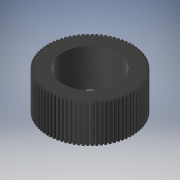
# Autodesk Inventor part: タミヤダンパー部品3
Saved by Autodesk Inventor 2020.1 (Build 241239000, 239)
## iProperties
Created: 2018-09-17
Part Number: タミヤダンパー部品3
Material: アセタール樹脂、黒
Document SubType Name: Modeling
Designer: 杉本　賢二郎
Density: 1.425 g/cm^3
Appearance: 滑らか - 黒
Author: 杉本　賢二郎
Autodesk Inventor part; units mm, degrees
ref_plane "YZ Plane" through (0, 0, 0) normal (1, 0, 0) x (0, 1, 0)
ref_plane "XZ Plane" through (0, 0, 0) normal (0, 1, 0) x (-1, 0, 0)
ref_plane "XY Plane" through (0, 0, 0) normal (0, 0, 1) x (1, 0, 0)
sketch "スケッチ1" plane through (0, 0, 0) normal (0, 1, 0) x (-1, 0, 0)
  arc A0 (0.0974, 4.9991) -> (-0.0974, 4.9991) centre (0, 0) ccw
  arc A1 (0.05, 4.8047) -> (-0.05, 4.8047) centre (0, 0) ccw
  line L0 (0.05, 4.8047) -> (0.0974, 4.9991)
  line L1 (-0.05, 4.8047) -> (-0.0974, 4.9991)
  line L2 (0, 4.9011) -> (0, 0)
  line L3 (-0.4268, 4.786) -> (-0.4893, 4.976)
  arc A2 (-0.2952, 4.9913) -> (-0.4893, 4.976) centre (0, 0) ccw
  line L4 (-0.3271, 4.7939) -> (-0.2952, 4.9913)
  arc A3 (-0.3271, 4.7939) -> (-0.4268, 4.786) centre (0, 0) ccw
  line L5 (-0.801, 4.7378) -> (-0.8782, 4.9223)
  arc A4 (-0.6859, 4.9527) -> (-0.8782, 4.9223) centre (0, 0) ccw
  line L6 (-0.7022, 4.7534) -> (-0.6859, 4.9527)
  arc A5 (-0.7022, 4.7534) -> (-0.801, 4.7378) centre (0, 0) ccw
  line L7 (-1.1703, 4.6603) -> (-1.2617, 4.8382)
  arc A6 (-1.0723, 4.8837) -> (-1.2617, 4.8382) centre (0, 0) ccw
  line L8 (-1.073, 4.6837) -> (-1.0723, 4.8837)
  arc A7 (-1.073, 4.6837) -> (-1.1703, 4.6603) centre (0, 0) ccw
  line L9 (-1.5323, 4.5541) -> (-1.6374, 4.7243)
  arc A8 (-1.4522, 4.7845) -> (-1.6374, 4.7243) centre (0, 0) ccw
  line L10 (-1.4372, 4.585) -> (-1.4522, 4.7845)
  arc A9 (-1.4372, 4.585) -> (-1.5323, 4.5541) centre (0, 0) ccw
  line L11 (-1.8849, 4.4199) -> (-2.003, 4.5813)
  arc A10 (-1.8231, 4.6558) -> (-2.003, 4.5813) centre (0, 0) ccw
  line L12 (-1.7925, 4.4581) -> (-1.8231, 4.6558)
  arc A11 (-1.7925, 4.4581) -> (-1.8849, 4.4199) centre (0, 0) ccw
  line L13 (-2.2259, 4.2584) -> (-2.3563, 4.41)
  arc A12 (-2.1828, 4.4984) -> (-2.3563, 4.41) centre (0, 0) ccw
  line L14 (-2.1368, 4.3038) -> (-2.1828, 4.4984)
  arc A13 (-2.1368, 4.3038) -> (-2.2259, 4.2584) centre (0, 0) ccw
  line L15 (-2.5531, 4.0706) -> (-2.695, 4.2115)
  arc A14 (-2.529, 4.3133) -> (-2.695, 4.2115) centre (0, 0) ccw
  line L16 (-2.4678, 4.1228) -> (-2.529, 4.3133)
  arc A15 (-2.4678, 4.1228) -> (-2.5531, 4.0706) centre (0, 0) ccw
  line L17 (-2.8646, 3.8577) -> (-3.0171, 3.9871)
  arc A16 (-2.8596, 4.1015) -> (-3.0171, 3.9871) centre (0, 0) ccw
  line L18 (-2.7837, 3.9165) -> (-2.8596, 4.1015)
  arc A17 (-2.7837, 3.9165) -> (-2.8646, 3.8577) centre (0, 0) ccw
  line L19 (-3.1584, 3.6211) -> (-3.3207, 3.7381)
  arc A18 (-3.1726, 3.8645) -> (-3.3207, 3.7381) centre (0, 0) ccw
  line L20 (-3.0824, 3.686) -> (-3.1726, 3.8645)
  arc A19 (-3.0824, 3.686) -> (-3.1584, 3.6211) centre (0, 0) ccw
  line L21 (-3.4328, 3.3621) -> (-3.6037, 3.466)
  arc A20 (-3.466, 3.6037) -> (-3.6037, 3.466) centre (0, 0) ccw
  line L22 (-3.3621, 3.4328) -> (-3.466, 3.6037)
  arc A21 (-3.3621, 3.4328) -> (-3.4328, 3.3621) centre (0, 0) ccw
  line L23 (-3.686, 3.0824) -> (-3.8645, 3.1726)
  arc A22 (-3.7381, 3.3207) -> (-3.8645, 3.1726) centre (0, 0) ccw
  line L24 (-3.6211, 3.1584) -> (-3.7381, 3.3207)
  arc A23 (-3.6211, 3.1584) -> (-3.686, 3.0824) centre (0, 0) ccw
  line L25 (-3.9165, 2.7837) -> (-4.1015, 2.8596)
  arc A24 (-3.9871, 3.0171) -> (-4.1015, 2.8596) centre (0, 0) ccw
  line L26 (-3.8577, 2.8646) -> (-3.9871, 3.0171)
  arc A25 (-3.8577, 2.8646) -> (-3.9165, 2.7837) centre (0, 0) ccw
  line L27 (-4.1228, 2.4678) -> (-4.3133, 2.529)
  arc A26 (-4.2115, 2.695) -> (-4.3133, 2.529) centre (0, 0) ccw
  line L28 (-4.0706, 2.5531) -> (-4.2115, 2.695)
  arc A27 (-4.0706, 2.5531) -> (-4.1228, 2.4678) centre (0, 0) ccw
  line L29 (-4.3038, 2.1368) -> (-4.4984, 2.1828)
  arc A28 (-4.41, 2.3563) -> (-4.4984, 2.1828) centre (0, 0) ccw
  line L30 (-4.2584, 2.2259) -> (-4.41, 2.3563)
  arc A29 (-4.2584, 2.2259) -> (-4.3038, 2.1368) centre (0, 0) ccw
  line L31 (-4.4581, 1.7925) -> (-4.6558, 1.8231)
  arc A30 (-4.5813, 2.003) -> (-4.6558, 1.8231) centre (0, 0) ccw
  line L32 (-4.4199, 1.8849) -> (-4.5813, 2.003)
  arc A31 (-4.4199, 1.8849) -> (-4.4581, 1.7925) centre (0, 0) ccw
  line L33 (-4.585, 1.4372) -> (-4.7845, 1.4522)
  arc A32 (-4.7243, 1.6374) -> (-4.7845, 1.4522) centre (0, 0) ccw
  line L34 (-4.5541, 1.5323) -> (-4.7243, 1.6374)
  arc A33 (-4.5541, 1.5323) -> (-4.585, 1.4372) centre (0, 0) ccw
  line L35 (-4.6837, 1.073) -> (-4.8837, 1.0723)
  arc A34 (-4.8382, 1.2617) -> (-4.8837, 1.0723) centre (0, 0) ccw
  line L36 (-4.6603, 1.1703) -> (-4.8382, 1.2617)
  arc A35 (-4.6603, 1.1703) -> (-4.6837, 1.073) centre (0, 0) ccw
  line L37 (-4.7534, 0.7022) -> (-4.9527, 0.6859)
  arc A36 (-4.9223, 0.8782) -> (-4.9527, 0.6859) centre (0, 0) ccw
  line L38 (-4.7378, 0.801) -> (-4.9223, 0.8782)
  arc A37 (-4.7378, 0.801) -> (-4.7534, 0.7022) centre (0, 0) ccw
  line L39 (-4.7939, 0.3271) -> (-4.9913, 0.2952)
  arc A38 (-4.976, 0.4893) -> (-4.9913, 0.2952) centre (0, 0) ccw
  line L40 (-4.786, 0.4268) -> (-4.976, 0.4893)
  arc A39 (-4.786, 0.4268) -> (-4.7939, 0.3271) centre (0, 0) ccw
  line L41 (-4.8047, -0.05) -> (-4.9991, -0.0974)
  arc A40 (-4.9991, 0.0974) -> (-4.9991, -0.0974) centre (0, 0) ccw
  line L42 (-4.8047, 0.05) -> (-4.9991, 0.0974)
  arc A41 (-4.8047, 0.05) -> (-4.8047, -0.05) centre (0, 0) ccw
  line L43 (-4.786, -0.4268) -> (-4.976, -0.4893)
  arc A42 (-4.9913, -0.2952) -> (-4.976, -0.4893) centre (0, 0) ccw
  line L44 (-4.7939, -0.3271) -> (-4.9913, -0.2952)
  arc A43 (-4.7939, -0.3271) -> (-4.786, -0.4268) centre (0, 0) ccw
  line L45 (-4.7378, -0.801) -> (-4.9223, -0.8782)
  arc A44 (-4.9527, -0.6859) -> (-4.9223, -0.8782) centre (0, 0) ccw
  line L46 (-4.7534, -0.7022) -> (-4.9527, -0.6859)
  arc A45 (-4.7534, -0.7022) -> (-4.7378, -0.801) centre (0, 0) ccw
  line L47 (-4.6603, -1.1703) -> (-4.8382, -1.2617)
  arc A46 (-4.8837, -1.0723) -> (-4.8382, -1.2617) centre (0, 0) ccw
  line L48 (-4.6837, -1.073) -> (-4.8837, -1.0723)
  arc A47 (-4.6837, -1.073) -> (-4.6603, -1.1703) centre (0, 0) ccw
  line L49 (-4.5541, -1.5323) -> (-4.7243, -1.6374)
  arc A48 (-4.7845, -1.4522) -> (-4.7243, -1.6374) centre (0, 0) ccw
  line L50 (-4.585, -1.4372) -> (-4.7845, -1.4522)
  arc A49 (-4.585, -1.4372) -> (-4.5541, -1.5323) centre (0, 0) ccw
  line L51 (-4.4199, -1.8849) -> (-4.5813, -2.003)
  arc A50 (-4.6558, -1.8231) -> (-4.5813, -2.003) centre (0, 0) ccw
  line L52 (-4.4581, -1.7925) -> (-4.6558, -1.8231)
  arc A51 (-4.4581, -1.7925) -> (-4.4199, -1.8849) centre (0, 0) ccw
  line L53 (-4.2584, -2.2259) -> (-4.41, -2.3563)
  arc A52 (-4.4984, -2.1828) -> (-4.41, -2.3563) centre (0, 0) ccw
  line L54 (-4.3038, -2.1368) -> (-4.4984, -2.1828)
  arc A53 (-4.3038, -2.1368) -> (-4.2584, -2.2259) centre (0, 0) ccw
  line L55 (-4.0706, -2.5531) -> (-4.2115, -2.695)
  arc A54 (-4.3133, -2.529) -> (-4.2115, -2.695) centre (0, 0) ccw
  line L56 (-4.1228, -2.4678) -> (-4.3133, -2.529)
  arc A55 (-4.1228, -2.4678) -> (-4.0706, -2.5531) centre (0, 0) ccw
  line L57 (-3.8577, -2.8646) -> (-3.9871, -3.0171)
  arc A56 (-4.1015, -2.8596) -> (-3.9871, -3.0171) centre (0, 0) ccw
  line L58 (-3.9165, -2.7837) -> (-4.1015, -2.8596)
  arc A57 (-3.9165, -2.7837) -> (-3.8577, -2.8646) centre (0, 0) ccw
  line L59 (-3.6211, -3.1584) -> (-3.7381, -3.3207)
  arc A58 (-3.8645, -3.1726) -> (-3.7381, -3.3207) centre (0, 0) ccw
  line L60 (-3.686, -3.0824) -> (-3.8645, -3.1726)
  arc A59 (-3.686, -3.0824) -> (-3.6211, -3.1584) centre (0, 0) ccw
  line L61 (-3.3621, -3.4328) -> (-3.466, -3.6037)
  arc A60 (-3.6037, -3.466) -> (-3.466, -3.6037) centre (0, 0) ccw
  line L62 (-3.4328, -3.3621) -> (-3.6037, -3.466)
  arc A61 (-3.4328, -3.3621) -> (-3.3621, -3.4328) centre (0, 0) ccw
  line L63 (-3.0824, -3.686) -> (-3.1726, -3.8645)
  arc A62 (-3.3207, -3.7381) -> (-3.1726, -3.8645) centre (0, 0) ccw
  line L64 (-3.1584, -3.6211) -> (-3.3207, -3.7381)
  arc A63 (-3.1584, -3.6211) -> (-3.0824, -3.686) centre (0, 0) ccw
  line L65 (-2.7837, -3.9165) -> (-2.8596, -4.1015)
  arc A64 (-3.0171, -3.9871) -> (-2.8596, -4.1015) centre (0, 0) ccw
  line L66 (-2.8646, -3.8577) -> (-3.0171, -3.9871)
  arc A65 (-2.8646, -3.8577) -> (-2.7837, -3.9165) centre (0, 0) ccw
  line L67 (-2.4678, -4.1228) -> (-2.529, -4.3133)
  arc A66 (-2.695, -4.2115) -> (-2.529, -4.3133) centre (0, 0) ccw
  line L68 (-2.5531, -4.0706) -> (-2.695, -4.2115)
  arc A67 (-2.5531, -4.0706) -> (-2.4678, -4.1228) centre (0, 0) ccw
  line L69 (-2.1368, -4.3038) -> (-2.1828, -4.4984)
  arc A68 (-2.3563, -4.41) -> (-2.1828, -4.4984) centre (0, 0) ccw
  line L70 (-2.2259, -4.2584) -> (-2.3563, -4.41)
  arc A69 (-2.2259, -4.2584) -> (-2.1368, -4.3038) centre (0, 0) ccw
  line L71 (-1.7925, -4.4581) -> (-1.8231, -4.6558)
  arc A70 (-2.003, -4.5813) -> (-1.8231, -4.6558) centre (0, 0) ccw
  line L72 (-1.8849, -4.4199) -> (-2.003, -4.5813)
  arc A71 (-1.8849, -4.4199) -> (-1.7925, -4.4581) centre (0, 0) ccw
  line L73 (-1.4372, -4.585) -> (-1.4522, -4.7845)
  arc A72 (-1.6374, -4.7243) -> (-1.4522, -4.7845) centre (0, 0) ccw
  line L74 (-1.5323, -4.5541) -> (-1.6374, -4.7243)
  arc A73 (-1.5323, -4.5541) -> (-1.4372, -4.585) centre (0, 0) ccw
  line L75 (-1.073, -4.6837) -> (-1.0723, -4.8837)
  arc A74 (-1.2617, -4.8382) -> (-1.0723, -4.8837) centre (0, 0) ccw
  line L76 (-1.1703, -4.6603) -> (-1.2617, -4.8382)
  arc A75 (-1.1703, -4.6603) -> (-1.073, -4.6837) centre (0, 0) ccw
  line L77 (-0.7022, -4.7534) -> (-0.6859, -4.9527)
  arc A76 (-0.8782, -4.9223) -> (-0.6859, -4.9527) centre (0, 0) ccw
  line L78 (-0.801, -4.7378) -> (-0.8782, -4.9223)
  arc A77 (-0.801, -4.7378) -> (-0.7022, -4.7534) centre (0, 0) ccw
  line L79 (-0.3271, -4.7939) -> (-0.2952, -4.9913)
  arc A78 (-0.4893, -4.976) -> (-0.2952, -4.9913) centre (0, 0) ccw
  line L80 (-0.4268, -4.786) -> (-0.4893, -4.976)
  arc A79 (-0.4268, -4.786) -> (-0.3271, -4.7939) centre (0, 0) ccw
  line L81 (0.05, -4.8047) -> (0.0974, -4.9991)
  arc A80 (-0.0974, -4.9991) -> (0.0974, -4.9991) centre (0, 0) ccw
  line L82 (-0.05, -4.8047) -> (-0.0974, -4.9991)
  arc A81 (-0.05, -4.8047) -> (0.05, -4.8047) centre (0, 0) ccw
  line L83 (0.4268, -4.786) -> (0.4893, -4.976)
  arc A82 (0.2952, -4.9913) -> (0.4893, -4.976) centre (0, 0) ccw
  line L84 (0.3271, -4.7939) -> (0.2952, -4.9913)
  arc A83 (0.3271, -4.7939) -> (0.4268, -4.786) centre (0, 0) ccw
  line L85 (0.801, -4.7378) -> (0.8782, -4.9223)
  arc A84 (0.6859, -4.9527) -> (0.8782, -4.9223) centre (0, 0) ccw
  line L86 (0.7022, -4.7534) -> (0.6859, -4.9527)
  arc A85 (0.7022, -4.7534) -> (0.801, -4.7378) centre (0, 0) ccw
  line L87 (1.1703, -4.6603) -> (1.2617, -4.8382)
  arc A86 (1.0723, -4.8837) -> (1.2617, -4.8382) centre (0, 0) ccw
  line L88 (1.073, -4.6837) -> (1.0723, -4.8837)
  arc A87 (1.073, -4.6837) -> (1.1703, -4.6603) centre (0, 0) ccw
  line L89 (1.5323, -4.5541) -> (1.6374, -4.7243)
  arc A88 (1.4522, -4.7845) -> (1.6374, -4.7243) centre (0, 0) ccw
  line L90 (1.4372, -4.585) -> (1.4522, -4.7845)
  arc A89 (1.4372, -4.585) -> (1.5323, -4.5541) centre (0, 0) ccw
  line L91 (1.8849, -4.4199) -> (2.003, -4.5813)
  arc A90 (1.8231, -4.6558) -> (2.003, -4.5813) centre (0, 0) ccw
  line L92 (1.7925, -4.4581) -> (1.8231, -4.6558)
  arc A91 (1.7925, -4.4581) -> (1.8849, -4.4199) centre (0, 0) ccw
  line L93 (2.2259, -4.2584) -> (2.3563, -4.41)
  arc A92 (2.1828, -4.4984) -> (2.3563, -4.41) centre (0, 0) ccw
  line L94 (2.1368, -4.3038) -> (2.1828, -4.4984)
  arc A93 (2.1368, -4.3038) -> (2.2259, -4.2584) centre (0, 0) ccw
  line L95 (2.5531, -4.0706) -> (2.695, -4.2115)
  arc A94 (2.529, -4.3133) -> (2.695, -4.2115) centre (0, 0) ccw
  line L96 (2.4678, -4.1228) -> (2.529, -4.3133)
  arc A95 (2.4678, -4.1228) -> (2.5531, -4.0706) centre (0, 0) ccw
  line L97 (2.8646, -3.8577) -> (3.0171, -3.9871)
  arc A96 (2.8596, -4.1015) -> (3.0171, -3.9871) centre (0, 0) ccw
  line L98 (2.7837, -3.9165) -> (2.8596, -4.1015)
  arc A97 (2.7837, -3.9165) -> (2.8646, -3.8577) centre (0, 0) ccw
  line L99 (3.1584, -3.6211) -> (3.3207, -3.7381)
  arc A98 (3.1726, -3.8645) -> (3.3207, -3.7381) centre (0, 0) ccw
  line L100 (3.0824, -3.686) -> (3.1726, -3.8645)
  arc A99 (3.0824, -3.686) -> (3.1584, -3.6211) centre (0, 0) ccw
  line L101 (3.4328, -3.3621) -> (3.6037, -3.466)
  arc A100 (3.466, -3.6037) -> (3.6037, -3.466) centre (0, 0) ccw
  line L102 (3.3621, -3.4328) -> (3.466, -3.6037)
  arc A101 (3.3621, -3.4328) -> (3.4328, -3.3621) centre (0, 0) ccw
  line L103 (3.686, -3.0824) -> (3.8645, -3.1726)
  arc A102 (3.7381, -3.3207) -> (3.8645, -3.1726) centre (0, 0) ccw
  line L104 (3.6211, -3.1584) -> (3.7381, -3.3207)
  arc A103 (3.6211, -3.1584) -> (3.686, -3.0824) centre (0, 0) ccw
  line L105 (3.9165, -2.7837) -> (4.1015, -2.8596)
  arc A104 (3.9871, -3.0171) -> (4.1015, -2.8596) centre (0, 0) ccw
  line L106 (3.8577, -2.8646) -> (3.9871, -3.0171)
  arc A105 (3.8577, -2.8646) -> (3.9165, -2.7837) centre (0, 0) ccw
  line L107 (4.1228, -2.4678) -> (4.3133, -2.529)
  arc A106 (4.2115, -2.695) -> (4.3133, -2.529) centre (0, 0) ccw
  line L108 (4.0706, -2.5531) -> (4.2115, -2.695)
  arc A107 (4.0706, -2.5531) -> (4.1228, -2.4678) centre (0, 0) ccw
  line L109 (4.3038, -2.1368) -> (4.4984, -2.1828)
  arc A108 (4.41, -2.3563) -> (4.4984, -2.1828) centre (0, 0) ccw
  line L110 (4.2584, -2.2259) -> (4.41, -2.3563)
  arc A109 (4.2584, -2.2259) -> (4.3038, -2.1368) centre (0, 0) ccw
  line L111 (4.4581, -1.7925) -> (4.6558, -1.8231)
  arc A110 (4.5813, -2.003) -> (4.6558, -1.8231) centre (0, 0) ccw
  line L112 (4.4199, -1.8849) -> (4.5813, -2.003)
  arc A111 (4.4199, -1.8849) -> (4.4581, -1.7925) centre (0, 0) ccw
  line L113 (4.585, -1.4372) -> (4.7845, -1.4522)
  arc A112 (4.7243, -1.6374) -> (4.7845, -1.4522) centre (0, 0) ccw
  line L114 (4.5541, -1.5323) -> (4.7243, -1.6374)
  arc A113 (4.5541, -1.5323) -> (4.585, -1.4372) centre (0, 0) ccw
  line L115 (4.6837, -1.073) -> (4.8837, -1.0723)
  arc A114 (4.8382, -1.2617) -> (4.8837, -1.0723) centre (0, 0) ccw
  line L116 (4.6603, -1.1703) -> (4.8382, -1.2617)
  arc A115 (4.6603, -1.1703) -> (4.6837, -1.073) centre (0, 0) ccw
  line L117 (4.7534, -0.7022) -> (4.9527, -0.6859)
  arc A116 (4.9223, -0.8782) -> (4.9527, -0.6859) centre (0, 0) ccw
  line L118 (4.7378, -0.801) -> (4.9223, -0.8782)
  arc A117 (4.7378, -0.801) -> (4.7534, -0.7022) centre (0, 0) ccw
  line L119 (4.7939, -0.3271) -> (4.9913, -0.2952)
  arc A118 (4.976, -0.4893) -> (4.9913, -0.2952) centre (0, 0) ccw
  line L120 (4.786, -0.4268) -> (4.976, -0.4893)
  arc A119 (4.786, -0.4268) -> (4.7939, -0.3271) centre (0, 0) ccw
  line L121 (4.8047, 0.05) -> (4.9991, 0.0974)
  arc A120 (4.9991, -0.0974) -> (4.9991, 0.0974) centre (0, 0) ccw
  line L122 (4.8047, -0.05) -> (4.9991, -0.0974)
  arc A121 (4.8047, -0.05) -> (4.8047, 0.05) centre (0, 0) ccw
  line L123 (4.786, 0.4268) -> (4.976, 0.4893)
  arc A122 (4.9913, 0.2952) -> (4.976, 0.4893) centre (0, 0) ccw
  line L124 (4.7939, 0.3271) -> (4.9913, 0.2952)
  arc A123 (4.7939, 0.3271) -> (4.786, 0.4268) centre (0, 0) ccw
  line L125 (4.7378, 0.801) -> (4.9223, 0.8782)
  arc A124 (4.9527, 0.6859) -> (4.9223, 0.8782) centre (0, 0) ccw
  line L126 (4.7534, 0.7022) -> (4.9527, 0.6859)
  arc A125 (4.7534, 0.7022) -> (4.7378, 0.801) centre (0, 0) ccw
  line L127 (4.6603, 1.1703) -> (4.8382, 1.2617)
  arc A126 (4.8837, 1.0723) -> (4.8382, 1.2617) centre (0, 0) ccw
  line L128 (4.6837, 1.073) -> (4.8837, 1.0723)
  arc A127 (4.6837, 1.073) -> (4.6603, 1.1703) centre (0, 0) ccw
  line L129 (4.5541, 1.5323) -> (4.7243, 1.6374)
  arc A128 (4.7845, 1.4522) -> (4.7243, 1.6374) centre (0, 0) ccw
  line L130 (4.585, 1.4372) -> (4.7845, 1.4522)
  arc A129 (4.585, 1.4372) -> (4.5541, 1.5323) centre (0, 0) ccw
  line L131 (4.4199, 1.8849) -> (4.5813, 2.003)
  arc A130 (4.6558, 1.8231) -> (4.5813, 2.003) centre (0, 0) ccw
  line L132 (4.4581, 1.7925) -> (4.6558, 1.8231)
  arc A131 (4.4581, 1.7925) -> (4.4199, 1.8849) centre (0, 0) ccw
  line L133 (4.2584, 2.2259) -> (4.41, 2.3563)
  arc A132 (4.4984, 2.1828) -> (4.41, 2.3563) centre (0, 0) ccw
  line L134 (4.3038, 2.1368) -> (4.4984, 2.1828)
  arc A133 (4.3038, 2.1368) -> (4.2584, 2.2259) centre (0, 0) ccw
  line L135 (4.0706, 2.5531) -> (4.2115, 2.695)
  arc A134 (4.3133, 2.529) -> (4.2115, 2.695) centre (0, 0) ccw
  line L136 (4.1228, 2.4678) -> (4.3133, 2.529)
  arc A135 (4.1228, 2.4678) -> (4.0706, 2.5531) centre (0, 0) ccw
  line L137 (3.8577, 2.8646) -> (3.9871, 3.0171)
  arc A136 (4.1015, 2.8596) -> (3.9871, 3.0171) centre (0, 0) ccw
  line L138 (3.9165, 2.7837) -> (4.1015, 2.8596)
  arc A137 (3.9165, 2.7837) -> (3.8577, 2.8646) centre (0, 0) ccw
  line L139 (3.6211, 3.1584) -> (3.7381, 3.3207)
  arc A138 (3.8645, 3.1726) -> (3.7381, 3.3207) centre (0, 0) ccw
  line L140 (3.686, 3.0824) -> (3.8645, 3.1726)
  arc A139 (3.686, 3.0824) -> (3.6211, 3.1584) centre (0, 0) ccw
  line L141 (3.3621, 3.4328) -> (3.466, 3.6037)
  arc A140 (3.6037, 3.466) -> (3.466, 3.6037) centre (0, 0) ccw
  line L142 (3.4328, 3.3621) -> (3.6037, 3.466)
  arc A141 (3.4328, 3.3621) -> (3.3621, 3.4328) centre (0, 0) ccw
  line L143 (3.0824, 3.686) -> (3.1726, 3.8645)
  arc A142 (3.3207, 3.7381) -> (3.1726, 3.8645) centre (0, 0) ccw
  line L144 (3.1584, 3.6211) -> (3.3207, 3.7381)
  arc A143 (3.1584, 3.6211) -> (3.0824, 3.686) centre (0, 0) ccw
  line L145 (2.7837, 3.9165) -> (2.8596, 4.1015)
  arc A144 (3.0171, 3.9871) -> (2.8596, 4.1015) centre (0, 0) ccw
  line L146 (2.8646, 3.8577) -> (3.0171, 3.9871)
  arc A145 (2.8646, 3.8577) -> (2.7837, 3.9165) centre (0, 0) ccw
  line L147 (2.4678, 4.1228) -> (2.529, 4.3133)
  arc A146 (2.695, 4.2115) -> (2.529, 4.3133) centre (0, 0) ccw
  line L148 (2.5531, 4.0706) -> (2.695, 4.2115)
  arc A147 (2.5531, 4.0706) -> (2.4678, 4.1228) centre (0, 0) ccw
  line L149 (2.1368, 4.3038) -> (2.1828, 4.4984)
  arc A148 (2.3563, 4.41) -> (2.1828, 4.4984) centre (0, 0) ccw
  line L150 (2.2259, 4.2584) -> (2.3563, 4.41)
  arc A149 (2.2259, 4.2584) -> (2.1368, 4.3038) centre (0, 0) ccw
  line L151 (1.7925, 4.4581) -> (1.8231, 4.6558)
  arc A150 (2.003, 4.5813) -> (1.8231, 4.6558) centre (0, 0) ccw
  line L152 (1.8849, 4.4199) -> (2.003, 4.5813)
  arc A151 (1.8849, 4.4199) -> (1.7925, 4.4581) centre (0, 0) ccw
  line L153 (1.4372, 4.585) -> (1.4522, 4.7845)
  arc A152 (1.6374, 4.7243) -> (1.4522, 4.7845) centre (0, 0) ccw
  line L154 (1.5323, 4.5541) -> (1.6374, 4.7243)
  arc A153 (1.5323, 4.5541) -> (1.4372, 4.585) centre (0, 0) ccw
  line L155 (1.073, 4.6837) -> (1.0723, 4.8837)
  arc A154 (1.2617, 4.8382) -> (1.0723, 4.8837) centre (0, 0) ccw
  line L156 (1.1703, 4.6603) -> (1.2617, 4.8382)
  arc A155 (1.1703, 4.6603) -> (1.073, 4.6837) centre (0, 0) ccw
  line L157 (0.7022, 4.7534) -> (0.6859, 4.9527)
  arc A156 (0.8782, 4.9223) -> (0.6859, 4.9527) centre (0, 0) ccw
  line L158 (0.801, 4.7378) -> (0.8782, 4.9223)
  arc A157 (0.801, 4.7378) -> (0.7022, 4.7534) centre (0, 0) ccw
  line L159 (0.3271, 4.7939) -> (0.2952, 4.9913)
  arc A158 (0.4893, 4.976) -> (0.2952, 4.9913) centre (0, 0) ccw
  line L160 (0.4268, 4.786) -> (0.4893, 4.976)
  arc A159 (0.4268, 4.786) -> (0.3271, 4.7939) centre (0, 0) ccw
  circle A160 centre (0, 0) radius 3.25
  circle A161 centre (0, 0) radius 5
  dimension "d2" = 0.2
  dimension "d3" = 0.2
  dimension "d4" = 0.1
  dimension "d5" = 9.61
  dimension "d6" = 0.05
  dimension "d7" = 360
  dimension "d8" = 6.5
  dimension "d9" = 10
  constraints: 322 end point, 320 point on circle, 162 centre point, 83 coincident, 1 vertical, 802 other
  measures "d2" distance of L1.start L1.end
  measures "d3" distance of L0.start L0.end
  measures "d4" distance of L0.start L1.start
  measures "d5" diameter of A1
  measures "d6" distance from line of L2 L1.start
  measures "d8" diameter of A160
  measures "d9" diameter of A161
extrude "押し出し1" add sketch "スケッチ1" along normal blind 4.5 contours A161 L159 A159 L160 L157 A157 L158 L155 A155 L156 L153 A153 L154 L151 A151 L152 L149 A149 L150 L147 A147 L148 L145 A145 L146 L143 A143 L144 L141 A141 L142 L139 A139 L140 L137 A137 L138 L135 A135 L136 L133 A133 L134 L131 A131 L132 L129 A129 L130 L127 A127 L128 L125 A125 L126 L123 A123 L124 L121 A121 L122 L119 A119 L120 L117 A117 L118 L115 A115 L116 L113 A113 L114 L111 A111 L112 L109 A109 L110 L107 A107 L108 L105 A105 L106 L103 A103 L104 L101 A101 L102 L99 A99 L100 L97 A97 L98 L95 A95 L96 L93 A93 L94 L91 A91 L92 L89 A89 L90 L87 A87 L88 L85 A85 L86 L83 A83 L84 L81 A81 L82 L79 A79 L80 L77 A77 L78 L75 A75 L76 L73 A73 L74 L71 A71 L72 L69 A69 L70 L67 A67 L68 L65 A65 L66 L63 A63 L64 L61 A61 L62 L59 A59 L60 L57 A57 L58 L55 A55 L56 L53 A53 L54 L51 A51 L52 L49 A49 L50 L47 A47 L48 L45 A45 L46 L43 A43 L44 L41 A41 L42 L39 A39 L40 L37 A37 L38 L35 A35 L36 L33 A33 L34 L31 A31 L32 L29 A29 L30 L27 A27 L28 L25 A25 L26 L23 A23 L24 L21 A21 L22 L19 A19 L20 L17 A17 L18 L15 A15 L16 L13 A13 L14 L11 A11 L12 L9 A9 L10 L7 A7 L8 L5 A5 L6 L3 A3 L4 L1 A1 L0
equation "\"d3\" = d2"
